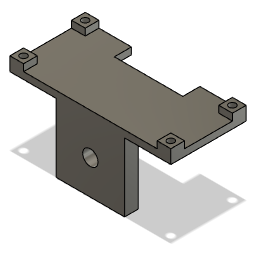
SupportUltraSons v1 (Autodesk Fusion 360 design; units mm, degrees)
Autodesk Fusion 360 part; units mm, degrees
sketch "Sketch1" plane through (0, 0, 0) normal (0, 1, 0) x (1, 0, 0)
  line L0 (-21.5, 9) -> (21.5, 9) construction
  line L1 (21.5, 9) -> (21.5, -9) construction
  line L2 (21.5, -9) -> (-21.5, -9) construction
  line L3 (-21.5, -9) -> (-21.5, 9) construction
  line L4 (-21.5, 9) -> (21.5, -9) construction
  circle A0 centre (-21.5, -9) radius 1
  circle A1 centre (21.5, -9) radius 1
  circle A2 centre (-21.5, 9) radius 1
  circle A3 centre (21.5, 9) radius 1
  line L5 (23.5, -11) -> (-23.5, -11)
  line L6 (-23.5, -11) -> (-23.5, 11)
  line L7 (-23.5, 11) -> (23.5, 11)
  line L8 (23.5, 11) -> (23.5, -11)
  line L9 (-23.5, 11) -> (-19.5, 11)
  line L10 (-19.5, 11) -> (-19.5, 7)
  line L11 (-19.5, 7) -> (-23.5, 7)
  line L12 (-23.5, 7) -> (-23.5, 11)
  line L13 (-23.5, -11) -> (-19.5, -11)
  line L14 (-19.5, -11) -> (-19.5, -7)
  line L15 (-19.5, -7) -> (-23.5, -7)
  line L16 (-23.5, -7) -> (-23.5, -11)
  line L17 (23.5, 11) -> (19.5, 11)
  line L18 (19.5, 11) -> (19.5, 7)
  line L19 (19.5, 7) -> (23.5, 7)
  line L20 (23.5, 7) -> (23.5, 11)
  line L21 (23.5, -11) -> (19.5, -11)
  line L22 (19.5, -11) -> (19.5, -7)
  line L23 (19.5, -7) -> (23.5, -7)
  line L24 (23.5, -7) -> (23.5, -11)
  line L25 (-10, 11) -> (10, 11)
  line L26 (10, 11) -> (10, 6)
  line L27 (10, 6) -> (-10, 6)
  line L28 (-10, 6) -> (-10, 11)
  dimension "d1" = 43
  dimension "d2" = 18
  dimension "d3" = 2
  dimension "d4" = 2
  dimension "d5" = 2
  dimension "d6" = 2
  dimension "d7" = -2
  dimension "d8" = 4
  dimension "d9" = 4
  dimension "d10" = 4
  dimension "d11" = 4
  dimension "d12" = 4
  dimension "d13" = 4
  dimension "d14" = 4
  dimension "d15" = 4
  dimension "d28" = 20
  dimension "d29" = 5
  constraint horizontal L0
  constraint vertical L1
  constraint horizontal L2
  constraint vertical L3
  constraint midpoint origin L4
  constraint coincident L2.end L3.start
  constraint coincident L1.end L2.start
  constraint coincident L0.start L3.end
  constraint coincident L0.end L1.start
  constraint horizontal L9
  constraint vertical L10
  constraint horizontal L11
  constraint vertical L12
  constraint horizontal L13
  constraint vertical L14
  constraint horizontal L15
  constraint vertical L16
  constraint horizontal L17
  constraint vertical L18
  constraint horizontal L19
  constraint vertical L20
  constraint horizontal L21
  constraint vertical L22
  constraint horizontal L23
  constraint vertical L24
  constraint horizontal L25
  constraint vertical L26
  constraint horizontal L27
  constraint vertical L28
  constraint coincident L7 L25.start
  constraint midpoint L7 L25
  measures "d1" distance of L0.start L0.end
  measures "d2" distance of L0.start L2.end
  measures "d3" diameter of A0
  measures "d4" diameter of A1
  measures "d5" diameter of A2
  measures "d6" diameter of A3
  measures "d8" distance of L6.end L9.end
  measures "d9" distance of L6.end L11.end
  measures "d10" distance of L5.end L13.end
  measures "d11" distance of L5.end L15.end
  measures "d12" distance of L7.end L17.end
  measures "d13" distance of L7.end L19.end
  measures "d14" distance of L5.start L21.end
  measures "d15" distance of L5.start L23.end
  measures "d28" distance of L25.start L25.end
  measures "d29" distance of L25.start L27.end
extrude "Extrude1" add sketch "Sketch1" against normal blind 2 contours L5 L8 L21 L22 L23 L24 | L5 L6 L7 L8 L10 L11 L14 L15 L18 L19 L22 L23 L26 L27 L28 | L5 L6 L13 L14 L15 L16 | L7 L8 L17 L18 L19 L20 | L6 L7 L9 L10 L11 L12
extrude "Extrude2" add sketch "Sketch1" along normal blind 2 contours L5 L8 L21 L22 L23 L24 | L5 L6 L13 L14 L15 L16 | L7 L8 L17 L18 L19 L20 | L6 L7 L9 L10 L11 L12
sketch "Sketch2" plane through (0, -2, 0) normal (0, -1, 0) x (1, 0, 0)
  circle A0 centre (-21.5, 9) radius 1
  circle A1 centre (-21.5, -9) radius 1
  circle A2 centre (21.5, 9) radius 1
  circle A3 centre (21.5, -9) radius 1
  line L0 (23.5, -11) -> (23.5, 11)
  line L1 (23.5, 11) -> (-23.5, 11)
  line L2 (-23.5, 11) -> (-23.5, -11)
  line L3 (10, -11) -> (23.5, -11)
  line L4 (-10, 11) -> (10, 11)
  line L5 (10, 11) -> (10, -9)
  line L6 (10, -9) -> (-10, -9)
  line L7 (-10, -9) -> (-10, 11)
  line L8 (23.5, 11) -> (-23.5, 11)
  line L9 (-10, 11) -> (10, 11)
  line L10 (10, 11) -> (10, 7)
  line L11 (10, 7) -> (-10, 7)
  line L12 (-10, 7) -> (-10, 11)
  line L13 (10, -6) -> (10, -11)
  line L14 (-23.5, -11) -> (-10, -11)
  line L15 (-10, -11) -> (-10, -6)
  line L16 (-10, -6) -> (10, -6)
  dimension "d20" = 20
  dimension "d21" = 20
  dimension "d22" = 4
  constraint horizontal L4
  constraint vertical L5
  constraint horizontal L6
  constraint vertical L7
  constraint coincident L1 L4.start
  constraint midpoint L4 L8
  constraint horizontal L9
  constraint vertical L10
  constraint horizontal L11
  constraint vertical L12
  constraint coincident L5 L10.end
  measures "d20" distance of L4.start L4.end
  measures "d21" distance of L4.start L6.end
  measures "d22" distance of L4.start L11.end
extrude "Extrude3" add sketch "Sketch2" along normal blind 20 contours L1 L4 L5 L7 L8 L9 L10 L11 L12
sketch "Sketch3" plane through (0, 0, 7) normal (0, 0, -1) x (-1, 0, 0)
  line L0 (10, -2) -> (-10, -2)
  line L1 (-10, -2) -> (-10, -22)
  line L2 (-10, -22) -> (10, -22)
  line L3 (10, -22) -> (10, -2)
  circle A0 centre (0, -12) radius 2.25
  line L4 (10, -22) -> (-10, -2) construction
  dimension "d25" = 4.5
  constraint coincident L2.end L3.start
  constraint coincident L0.end L1.start
  constraint midpoint A0.centre L4
  measures "d25" diameter of A0
extrude "Extrude4" cut sketch "Sketch3" against normal blind 4 contours A0
named bodies: "SupportUltraSon"
